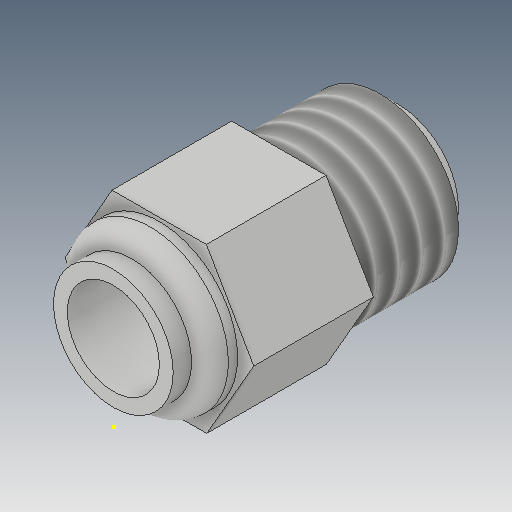
# Autodesk Inventor part: Pushfit-Adapter
Saved by Autodesk Inventor 2017 (Build 210142000, 142)
## iProperties
Created: 2016-07-07
Part Number: Pushfit-Adapter
Material: Generic
Document SubType Name: Modeling
Designer: joshmamo
Density: 1 g/cm^3
Appearance: Default
Mass: 0.608999 g
Surface Area: 7.45955 cm^2
Volume: 0.608999 cm^3
Author: joshmamo
Autodesk Inventor part; units mm, degrees
ref_plane "YZ Plane" through (0, 0, 0) normal (1, 0, 0) x (0, 1, 0)
ref_plane "XZ Plane" through (0, 0, 0) normal (0, 1, 0) x (-1, 0, 0)
ref_plane "XY Plane" through (0, 0, 0) normal (0, 0, 1) x (1, 0, 0)
sketch "Sketch1" plane through (0, 0, 0) normal (0, 0, 1) x (1, 0, 0)
  circle A0 centre (-0.0091, 4.1481) radius 4.25 projected
  point P0 (0, 0)
extrude "Extrusion1" add sketch "Sketch1" against normal blind 6.5
thread "Thread1" size "M9x1.25" class "6g" standard "ANSI Metric M Profile" full length
sketch "Sketch2" plane through (-0.0091, 4.1481, 0) normal (0, 0, 1) x (1, 0, 0)
  line L0 (2.5727, -4.4349) -> (-2.5544, -4.4455)
  line L1 (-2.5544, -4.4455) -> (-5.1271, -0.0106)
  line L2 (-5.1271, -0.0106) -> (-2.5727, 4.4349)
  line L3 (-2.5727, 4.4349) -> (2.5544, 4.4455)
  line L4 (2.5544, 4.4455) -> (5.1271, 0.0106)
  line L5 (5.1271, 0.0106) -> (2.5727, -4.4349)
  point P0 (0.0091, -4.1481)
  point P1 (0, 0)
  constraints: 12 end point, 13 other
extrude "Extrusion2" add sketch "Sketch2" along normal blind 6.5
sketch "Sketch3" plane through (-0.0091, 4.1481, 6.5) normal (0, 0, 1) x (1, 0, 0)
  circle A0 centre (0, 0) radius 4.25
  point P0 (0.0091, -4.1481)
  constraints: 1 centre point
extrude "Extrusion3" add sketch "Sketch3" along normal blind 1.5
fillet "Fillet1" radius 1 1 edges at (-4.2591, 4.1481, 8)
sketch "Sketch4" plane through (-0.0091, 4.1481, 8) normal (0, 0, 1) x (1, 0, 0)
  circle A0 centre (0, 0) radius 3.25
  point P0 (0.0091, -4.1481)
  constraints: 1 centre point
extrude "Extrusion4" add sketch "Sketch4" along normal blind 1
sketch "Sketch5" plane through (-0.0091, 4.1481, 9) normal (0, 0, 1) x (1, 0, 0)
  point P0 (0.0091, -4.1481)
sketch "Sketch6" plane through (-0.0091, 4.1481, 9) normal (0, 0, 1) x (1, 0, 0)
  circle A0 centre (0, 0) radius 3.25 projected
  circle A1 centre (0, 0) radius 2.5
  point P0 (0.0091, -4.1481)
  dimension "d11" = 5
  constraints: 1 centre point, 1 coincident
  measures "d11" diameter of A1
extrude "Extrusion5" cut sketch "Sketch6" against normal through all contours A1
chamfer "Chamfer1" distance 1 angle 45 1 edges at (-4.2591, 4.1481, -6.5)
body "Solid1"
